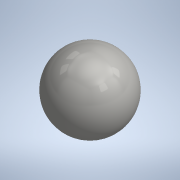
# Autodesk Inventor part: Rueda
Saved by Autodesk Inventor 2022.1 (Build 261234000, 234)
## iProperties
Part Number: Rueda
Material: Genérico
Document SubType Name: Modelado
Designer: seb_0
Appearance: Acero
Author: seb_0
Autodesk Inventor part; units mm, degrees
ref_plane "Plano YZ" through (0, 0, 0) normal (1, 0, 0) x (0, 1, 0)
ref_plane "Plano XZ" through (0, 0, 0) normal (0, 1, 0) x (-1, 0, 0)
ref_plane "Plano XY" through (0, 0, 0) normal (0, 0, 1) x (1, 0, 0)
sketch "Boceto1" plane through (0, 0, 0) normal (1, 0, 0) x (0, 1, 0)
  arc A0 (50.8, 0) -> (0, 0) centre (25.4, 0) ccw
  line L0 (50.8, 0) -> (0, 0)
  dimension "d0" = 50.8
  dimension "d1" = 25.4
  constraints: 2 end point, 2 point on circle, 1 centre point, 1 horizontal
  measures "d0" distance of L0.end L0.start
  measures "d1" radius of A0
revolve "Revolución1" add sketch "Boceto1" angle 360 about axis through (0, 50.8, 0) along (0, -1, 0)
